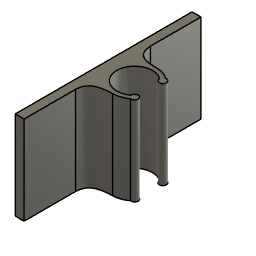
_Pen Holder Prototype.81b64bac-0799-4906-a694-e2d1f3394e13 (Autodesk Fusion 360 design; units mm, degrees)
Autodesk Fusion 360 part; units mm, degrees
sketch "Sketch1" plane through (0, 0, 0) normal (0, 1, 0) x (1, 0, 0)
  arc A0 (1.7813, 4.6719) -> (1.7813, -4.6719) centre (0, 0) ccw
  arc A1 (1.2375, 3.8563) -> (1.2375, -3.8563) centre (0, 0) ccw
  circle A2 centre (3.2, 3.2) radius 0.8
  line L0 (2.5, 0) -> (20, 0)
  circle A3 centre (3.2, -3.2) radius 0.8
  arc A4 (3.2606, 2.4023) -> (3.2606, -2.4023) centre (0, 0) ccw
  arc A5 (3.9807, 3.0255) -> (3.9807, -3.0255) centre (0, 0) ccw
  dimension "d4" = 5
  constraint concentric A1 A4
  constraint concentric A4 A5
  constraint symmetric A2 L0 A3
  constraint coincident A3 A4.end
  constraint coincident A3 A5.end
  constraint coincident A2 A4.start
  constraint coincident A2 A5.start
  measures "d4" radius of A0
extrude "Extrude1" add sketch "Sketch1" along normal blind 10 makes body 1
sketch "Sketch2" plane through (0, 0, 0) normal (1, 0, 0) x (0, 0, -1)
  line L0 (20, 10) -> (-20, 10)
  line L1 (-20, 10) -> (-20, -10)
  line L2 (-20, -10) -> (20, -10)
  line L3 (20, -10) -> (20, 10)
  line L4 (20, 10) -> (-20, -10) construction
  line L5 (-20, 10) -> (20, -10) construction
  dimension "d20" = 40
  dimension "d21" = 20
  constraint horizontal L0
  constraint perpendicular L0 L1
  constraint parallel L0 L2
  constraint parallel L1 L3
  constraint coincident L4 origin
  constraint coincident L5 origin
  measures "d20" distance of L1.end L2.end
  measures "d21" distance of L0.end L1.end
move_body "Move1" bodies 1 to x (1, 0, 0) y (0, 1, 0) z (0, 0, 1) at (5, 0, 0)
extrude "Extrude3" add sketch "Sketch2" against normal blind 2 separate body makes body 2
sketch "Sketch3" plane through (0, 10, 0) normal (0, 1, 0) x (-1, 0, 0)
  line L0 (0, 20) -> (0, -20)
  line L1 (0, -20) -> (2, -20)
  line L2 (2, -20) -> (2, 20)
  line L3 (2, 20) -> (0, 20)
  spline S0 degree 5 poles (-5, 5) (-4.8035, 5.004) (-4.4185, 5.0174) (-3.8655, 5.0543) (-3.1777, 5.1374) (-2.4065, 5.3019) (-1.7325, 5.5329) (-1.1655, 5.8372) (-0.7131, 6.2199) (-0.375, 6.681) (-0.1446, 7.2157) (-0.0401, 7.6981) (-0.0039, 8.0889) (0.0018, 8.362) (0, 8.5017) knots 0 0 0 0 0 0 0.1 0.2 0.3 0.4 0.5 0.6 0.7 0.8 0.9 1 1 1 1 1 1
  spline S1 degree 5 poles (-5, -5) (-4.7917, -4.9918) (-4.3843, -4.9839) (-3.8014, -4.9975) (-3.0812, -5.0673) (-2.2827, -5.2467) (-1.5952, -5.5267) (-1.0284, -5.9162) (-0.5886, -6.4208) (-0.2721, -7.0371) (-0.0701, -7.7572) (0.0071, -8.4097) (0.0206, -8.9394) (0.0101, -9.3102) (0, -9.5) knots 0 0 0 0 0 0 0.1 0.2 0.3 0.4 0.5 0.6 0.7 0.8 0.9 1 1 1 1 1 1
  spline S2 degree 5 poles (0, -9.5) (0, -9.1191) (0, -8.3592) (0, -7.2248) (0, -5.7231) (0, -3.8656) (0, -2.0294) (0, -0.2163) (0, 1.5723) (0, 3.3372) (0, 5.0801) (0, 6.4582) (0, 7.4832) (0, 8.1628) (0, 8.5017) knots 0 0 0 0 0 0 0.1 0.2 0.3 0.4 0.5 0.6 0.7 0.8 0.9 1 1 1 1 1 1
  arc A0 (-5, -5) -> (-5, 5) centre (-5, 0) ccw
  arc A1 (-7.4023, -3.2606) -> (-8.0255, -3.9807) centre (-8.2, -3.2) ccw
  arc A2 (-8.0255, -3.9807) -> (-8.0255, 3.9807) centre (-5, 0) ccw
  arc A3 (-8.0255, 3.9807) -> (-7.4023, 3.2606) centre (-8.2, 3.2) ccw
  arc A4 (-7.4023, -3.2606) -> (-7.4023, 3.2606) centre (-5, 0) ccw
  point P0 (-1, 6)
  point P1 (-1, -6)
  constraint coincident L0 S0.end
  constraint coincident L0 S1.end
  constraint coincident origin A0
  constraint tangent L0 A0
extrude "Extrude4" add sketch "Sketch3" against normal blind 20 contours L0 S0 S2 A0 A2 | L0 S1 S2 A0 A2 bodies 1 2
extrude "Extrude6" add 1 faces at (8.3891, 0, 3.1663) along direction (0, -1, 0) blind 10 on bodies 1 bodies 1
